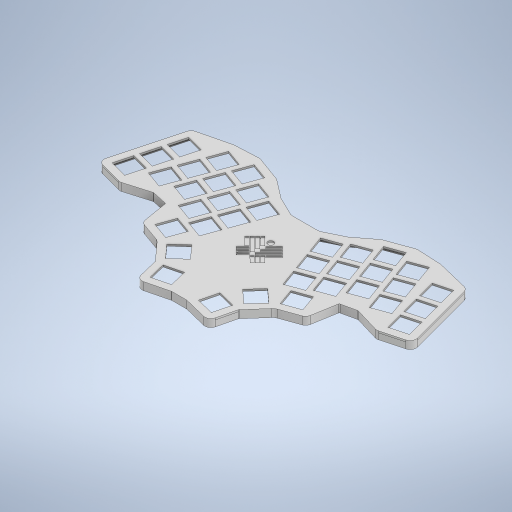
# Autodesk Inventor part: top
Saved by Autodesk Inventor 2024 (Build 280153000, 153)
## iProperties
Created: 2024-10-27
Part Number: top
Material: Generisch
Document SubType Name: Modeling
Designer: nikla
Density: 1 g/cm^3
Appearance: Vorgabe
Author: nikla
Autodesk Inventor part; units mm, degrees
(part 1 of 2)
ref_plane "YZ Plane" through (0, 0, 0) normal (1, 0, 0) x (0, 1, 0)
ref_plane "XZ Plane" through (0, 0, 0) normal (0, 1, 0) x (-1, 0, 0)
ref_plane "XY Plane" through (0, 0, 0) normal (0, 0, 1) x (1, 0, 0)
sketch "Skizze3" plane through (0, 0, 0) normal (0, 0, 1) x (1, 0, 0)
  line L0 (33.2927, 55.6855) -> (15.6286, 55.6855) projected
  line L1 (11.8229, 56.0361) -> (-3.9316, 63.7231) projected
  line L2 (37.0985, 56.0361) -> (52.8529, 63.7231) projected
  arc A0 (69.5641, 76.2372) -> (68.2289, 75.5042) centre (71.2739, 71.5396) ccw projected
  arc A1 (91.9431, 83.9654) -> (89.9858, 83.67) centre (91.6959, 78.9716) ccw projected
  arc A2 (112.5928, 82.8509) -> (111.6421, 82.9904) centre (111.3949, 77.9956) ccw projected
  arc A3 (141.8721, 73.0196) -> (138.2304, 76.582) centre (137.0429, 71.7256) ccw projected
  line L3 (141.8721, 73.0196) -> (156.3724, 18.9046) projected
  arc A4 (152.837, 12.781) -> (156.3724, 18.9046) centre (151.5429, 17.6106) ccw projected
  line L4 (152.837, 12.781) -> (134.5249, 7.8743) projected
  line L5 (131.8222, 7.9065) -> (111.3881, 13.9074) projected
  arc A5 (131.8222, 7.9065) -> (134.5249, 7.8743) centre (133.2309, 12.7036) ccw projected
  line L6 (110.8785, 13.9276) -> (98.6315, 11.2116) projected
  line L7 (97.8626, 10.4048) -> (94.4059, -9.7209) projected
  line L8 (91.1608, -13.5829) -> (75.8602, -19.0515) projected
  line L9 (59.9635, -35.5881) -> (72.8683, -21.2559) projected
  line L10 (55.8813, -51.867) -> (59.7317, -36.0348) projected
  line L11 (30.9758, -50.8402) -> (49.8133, -55.5369) projected
  arc A6 (49.8133, -55.5369) -> (55.8813, -51.867) centre (51.0229, -50.6854) ccw projected
  line L12 (18.202, -50.8106) -> (30.7193, -50.8106) projected
  line L13 (-0.892, -55.5369) -> (17.9455, -50.8402) projected
  arc A7 (-6.96, -51.867) -> (-0.892, -55.5369) centre (-2.1016, -50.6854) ccw projected
  line L14 (-10.8104, -36.0348) -> (-6.96, -51.867) projected
  line L15 (-23.947, -21.2559) -> (-11.0422, -35.5881) projected
  line L16 (-42.2395, -13.5829) -> (-26.9389, -19.0515) projected
  line L17 (-48.9413, 10.4048) -> (-45.4846, -9.7209) projected
  arc A8 (-45.4846, -9.7209) -> (-42.2395, -13.5829) centre (-40.5566, -8.8744) ccw projected
  line L18 (-61.9572, 13.9276) -> (-49.7102, 11.2116) projected
  line L19 (-82.9009, 7.9065) -> (-62.4668, 13.9074) projected
  line L20 (-103.9157, 12.781) -> (-85.6036, 7.8743) projected
  arc A9 (-107.4511, 18.9046) -> (-103.9157, 12.781) centre (-102.6216, 17.6106) ccw projected
  line L21 (-92.9508, 73.0196) -> (-107.4511, 18.9046) projected
  line L22 (-63.6715, 82.8509) -> (-89.3091, 76.582) projected
  arc A10 (-89.3091, 76.582) -> (-92.9508, 73.0196) centre (-88.1216, 71.7256) ccw projected
  line L23 (-4.112, 63.8334) -> (-19.3076, 75.5043) projected
  line L24 (-20.6428, 76.2372) -> (-41.0645, 83.67) projected
  line L25 (-43.0218, 83.9654) -> (-62.7208, 82.9904) projected
  line L26 (53.0333, 63.8334) -> (68.2289, 75.5043) projected
  line L27 (69.5641, 76.2372) -> (89.9858, 83.67) projected
  line L28 (91.9431, 83.9654) -> (111.6421, 82.9904) projected
  line L29 (112.5928, 82.8509) -> (138.2304, 76.582) projected
  line L30 (-82.1125, 32.7172) -> (-96.6013, 36.5996) projected
  line L31 (-96.6013, 36.5996) -> (-92.719, 51.0885) projected
  line L32 (-92.719, 51.0885) -> (-78.2301, 47.2061) projected
  line L33 (-78.2301, 47.2061) -> (-82.1125, 32.7172) projected
  line L34 (-31.0217, 57.7735) -> (-45.117, 62.9038) projected
  line L35 (-45.117, 62.9038) -> (-39.9867, 76.9992) projected
  line L36 (-39.9867, 76.9992) -> (-25.8914, 71.8689) projected
  line L37 (-25.8914, 71.8689) -> (-31.0217, 57.7735) projected
  line L38 (-16.5877, 41.8782) -> (-21.718, 27.7828) projected
  line L39 (-21.718, 27.7828) -> (-35.8134, 32.9131) projected
  line L40 (-35.8134, 32.9131) -> (-30.6831, 47.0085) projected
  line L41 (-30.6831, 47.0085) -> (-16.5877, 41.8782) projected
  line L42 (-20.0113, 20.7765) -> (-5.916, 15.6462) projected
  line L43 (-5.916, 15.6462) -> (-11.0463, 1.5508) projected
  line L44 (-11.0463, 1.5508) -> (-25.1417, 6.6811) projected
  line L45 (-25.1417, 6.6811) -> (-20.0113, 20.7765) projected
  line L46 (-4.5479, 19.405) -> (-18.6433, 24.5353) projected
  line L47 (-18.6433, 24.5353) -> (-13.513, 38.6307) projected
  line L48 (-13.513, 38.6307) -> (0.5824, 33.5004) projected
  line L49 (0.5824, 33.5004) -> (-4.5479, 19.405) projected
  line L50 (-10.0893, 59.7323) -> (-15.2196, 45.6369) projected
  line L51 (-15.2196, 45.6369) -> (-29.315, 50.7672) projected
  line L52 (-29.315, 50.7672) -> (-24.1847, 64.8626) projected
  line L53 (-24.1847, 64.8626) -> (-10.0893, 59.7323) projected
  line L54 (-59.4784, 35.1414) -> (-64.6087, 21.046) projected
  line L55 (-64.6087, 21.046) -> (-78.7041, 26.1763) projected
  line L56 (-78.7041, 26.1763) -> (-73.5738, 40.2717) projected
  line L57 (-73.5738, 40.2717) -> (-59.4784, 35.1414) projected
  line L58 (-77.1948, 51.0698) -> (-91.6837, 54.9522) projected
  line L59 (-91.6837, 54.9522) -> (-87.8013, 69.441) projected
  line L60 (-87.8013, 69.441) -> (-73.3125, 65.5587) projected
  line L61 (-73.3125, 65.5587) -> (-77.1948, 51.0698) projected
  line L62 (-46.4817, 70.8497) -> (-51.612, 56.7543) projected
  line L63 (-51.612, 56.7543) -> (-65.7074, 61.8846) projected
  line L64 (-65.7074, 61.8846) -> (-60.5771, 75.98) projected
  line L65 (-60.5771, 75.98) -> (-46.4817, 70.8497) projected
  line L66 (-37.52, 39.9193) -> (-51.6154, 45.0496) projected
  line L67 (-51.6154, 45.0496) -> (-46.4851, 59.145) projected
  line L68 (-46.4851, 59.145) -> (-32.3897, 54.0147) projected
  line L69 (-32.3897, 54.0147) -> (-37.52, 39.9193) projected
  line L70 (-37.1815, 29.1543) -> (-23.0861, 24.024) projected
  line L71 (-23.0861, 24.024) -> (-28.2164, 9.9286) projected
  line L72 (-28.2164, 9.9286) -> (-42.3118, 15.0589) projected
  line L73 (-42.3118, 15.0589) -> (-37.1815, 29.1543) projected
  line L74 (-33.1433, 5.2903) -> (-19.0184, 0.2419) projected
  line L75 (-19.0184, 0.2419) -> (-24.0668, -13.883) projected
  line L76 (-24.0668, -13.883) -> (-38.1917, -8.8346) projected
  line L77 (-38.1917, -8.8346) -> (-33.1433, 5.2903) projected
  line L78 (1.9505, 37.2592) -> (-12.1449, 42.3895) projected
  line L79 (-12.1449, 42.3895) -> (-7.0146, 56.4848) projected
  line L80 (-7.0146, 56.4848) -> (7.0808, 51.3545) projected
  line L81 (7.0808, 51.3545) -> (1.9505, 37.2592) projected
  line L82 (-52.9835, 41.2908) -> (-38.8881, 36.1605) projected
  line L83 (-38.8881, 36.1605) -> (-44.0184, 22.0651) projected
  line L84 (-44.0184, 22.0651) -> (-58.1138, 27.1954) projected
  line L85 (-58.1138, 27.1954) -> (-52.9835, 41.2908) projected
  line L86 (-52.9801, 52.9955) -> (-58.1104, 38.9001) projected
  line L87 (-58.1104, 38.9001) -> (-72.2057, 44.0304) projected
  line L88 (-72.2057, 44.0304) -> (-67.0754, 58.1258) projected
  line L89 (-67.0754, 58.1258) -> (-52.9801, 52.9955) projected
  line L90 (-97.6366, 32.7359) -> (-83.1478, 28.8535) projected
  line L91 (-83.1478, 28.8535) -> (-87.0301, 14.3647) projected
  line L92 (-87.0301, 14.3647) -> (-101.519, 18.247) projected
  line L93 (-101.519, 18.247) -> (-97.6366, 32.7359) projected
  arc A11 (-85.086, 9.8061) -> (-83.4644, 9.8255) centre (-84.3096, 12.7036) ccw projected
  line L94 (-63.0418, 15.823) -> (-83.4644, 9.8255) projected
  arc A12 (-61.5241, 15.8802) -> (-63.0418, 15.8229) centre (-62.1736, 12.9516) ccw projected
  line L95 (-49.2771, 13.1641) -> (-61.5241, 15.8802) projected
  arc A13 (-46.9702, 10.7433) -> (-49.2771, 13.1641) centre (-49.9266, 10.2356) ccw projected
  line L96 (-43.5135, -9.3823) -> (-46.9702, 10.7433) projected
  arc A14 (-43.5135, -9.3823) -> (-41.5663, -11.6996) centre (-40.5566, -8.8744) ccw projected
  line L97 (-26.2657, -17.1682) -> (-41.5663, -11.6996) projected
  arc A15 (-26.2657, -17.1682) -> (-25.1373, -16.9454) centre (-25.8881, -16.1115) ccw projected
  line L98 (-10.1529, -3.4534) -> (-25.1373, -16.9454) projected
  line L99 (10.8605, 54.2803) -> (-10.1529, -3.4534) projected
  line L100 (-4.7986, 61.9207) -> (10.8605, 54.2803) projected
  arc A16 (-5.3302, 62.2473) -> (-4.7986, 61.9208) centre (-3.5036, 64.6256) ccw projected
  line L101 (-20.5258, 73.9181) -> (-5.3302, 62.2473) projected
  arc A17 (-20.5258, 73.9181) -> (-21.3269, 74.3578) centre (-22.3526, 71.5396) ccw projected
  line L102 (-41.7486, 81.7906) -> (-21.3269, 74.3578) projected
  arc A18 (-41.7486, 81.7906) -> (-42.9229, 81.9679) centre (-42.7746, 78.9716) ccw projected
  line L103 (-62.622, 80.9928) -> (-42.9229, 81.9679) projected
  arc A19 (-62.622, 80.9928) -> (-63.1944, 80.9086) centre (-62.4736, 77.9956) ccw projected
  line L104 (-88.8341, 74.6393) -> (-63.1944, 80.9086) projected
  arc A20 (-88.8341, 74.6393) -> (-91.019, 72.5019) centre (-88.1216, 71.7256) ccw projected
  line L105 (-105.5193, 18.387) -> (-91.019, 72.5019) projected
  arc A21 (-105.5193, 18.387) -> (-103.398, 14.7129) centre (-102.6216, 17.6106) ccw projected
  line L106 (-85.086, 9.8061) -> (-103.398, 14.7129) projected
  line L107 (131.0338, 32.7172) -> (145.5226, 36.5996) projected
  line L108 (127.1514, 47.2061) -> (131.0338, 32.7172) projected
  line L109 (141.6403, 51.0885) -> (127.1514, 47.2061) projected
  line L110 (145.5226, 36.5996) -> (141.6403, 51.0885) projected
  line L111 (79.943, 57.7735) -> (94.0383, 62.9038) projected
  line L112 (74.8127, 71.8689) -> (79.943, 57.7735) projected
  line L113 (88.908, 76.9992) -> (74.8127, 71.8689) projected
  line L114 (94.0383, 62.9038) -> (88.908, 76.9992) projected
  line L115 (65.509, 41.8782) -> (70.6393, 27.7828) projected
  line L116 (79.6044, 47.0085) -> (65.509, 41.8782) projected
  line L117 (84.7347, 32.9131) -> (79.6044, 47.0085) projected
  line L118 (70.6393, 27.7828) -> (84.7347, 32.9131) projected
  line L119 (68.9327, 20.7765) -> (54.8373, 15.6462) projected
  line L120 (74.063, 6.6811) -> (68.9327, 20.7765) projected
  line L121 (59.9676, 1.5508) -> (74.063, 6.6811) projected
  line L122 (54.8373, 15.6462) -> (59.9676, 1.5508) projected
  line L123 (53.4692, 19.405) -> (67.5646, 24.5353) projected
  line L124 (48.3389, 33.5004) -> (53.4692, 19.405) projected
  line L125 (62.4343, 38.6307) -> (48.3389, 33.5004) projected
  line L126 (67.5646, 24.5353) -> (62.4343, 38.6307) projected
  line L127 (59.0106, 59.7323) -> (64.1409, 45.6369) projected
  line L128 (73.106, 64.8626) -> (59.0106, 59.7323) projected
  line L129 (78.2363, 50.7672) -> (73.106, 64.8626) projected
  line L130 (64.1409, 45.6369) -> (78.2363, 50.7672) projected
  line L131 (108.3997, 35.1414) -> (113.53, 21.046) projected
  line L132 (122.4951, 40.2717) -> (108.3997, 35.1414) projected
  line L133 (127.6254, 26.1763) -> (122.4951, 40.2717) projected
  line L134 (113.53, 21.046) -> (127.6254, 26.1763) projected
  line L135 (126.1161, 51.0698) -> (140.605, 54.9522) projected
  line L136 (122.2338, 65.5587) -> (126.1161, 51.0698) projected
  line L137 (136.7226, 69.441) -> (122.2338, 65.5587) projected
  line L138 (140.605, 54.9522) -> (136.7226, 69.441) projected
  line L139 (95.403, 70.8497) -> (100.5333, 56.7543) projected
  line L140 (109.4984, 75.98) -> (95.403, 70.8497) projected
  line L141 (114.6287, 61.8846) -> (109.4984, 75.98) projected
  line L142 (100.5333, 56.7543) -> (114.6287, 61.8846) projected
  line L143 (86.4413, 39.9193) -> (100.5367, 45.0496) projected
  line L144 (81.311, 54.0147) -> (86.4413, 39.9193) projected
  line L145 (95.4064, 59.145) -> (81.311, 54.0147) projected
  line L146 (100.5367, 45.0496) -> (95.4064, 59.145) projected
  line L147 (86.1028, 29.1543) -> (72.0074, 24.024) projected
  line L148 (91.2331, 15.0589) -> (86.1028, 29.1543) projected
  line L149 (77.1377, 9.9286) -> (91.2331, 15.0589) projected
  line L150 (72.0074, 24.024) -> (77.1377, 9.9286) projected
  line L151 (82.0646, 5.2903) -> (67.9397, 0.2419) projected
  line L152 (87.113, -8.8346) -> (82.0646, 5.2903) projected
  line L153 (72.9881, -13.883) -> (87.113, -8.8346) projected
  line L154 (67.9397, 0.2419) -> (72.9881, -13.883) projected
  line L155 (46.9708, 37.2592) -> (61.0662, 42.3895) projected
  line L156 (41.8405, 51.3545) -> (46.9708, 37.2592) projected
  line L157 (55.9359, 56.4848) -> (41.8405, 51.3545) projected
  line L158 (61.0662, 42.3895) -> (55.9359, 56.4848) projected
  line L159 (101.9048, 41.2908) -> (87.8094, 36.1605) projected
  line L160 (107.0351, 27.1954) -> (101.9048, 41.2908) projected
  line L161 (92.9397, 22.0651) -> (107.0351, 27.1954) projected
  line L162 (87.8094, 36.1605) -> (92.9397, 22.0651) projected
  line L163 (101.9014, 52.9955) -> (107.0317, 38.9001) projected
  line L164 (115.9967, 58.1258) -> (101.9014, 52.9955) projected
  line L165 (121.1271, 44.0304) -> (115.9967, 58.1258) projected
  line L166 (107.0317, 38.9001) -> (121.1271, 44.0304) projected
  line L167 (146.5579, 32.7359) -> (132.0691, 28.8535) projected
  line L168 (150.4403, 18.247) -> (146.5579, 32.7359) projected
  line L169 (135.9514, 14.3647) -> (150.4403, 18.247) projected
  line L170 (132.0691, 28.8535) -> (135.9514, 14.3647) projected
  arc A22 (132.3857, 9.8255) -> (134.0073, 9.8061) centre (133.2309, 12.7036) ccw projected
  line L171 (134.0073, 9.8061) -> (152.3194, 14.7129) projected
  arc A23 (152.3194, 14.7129) -> (154.4406, 18.387) centre (151.5429, 17.6106) ccw projected
  line L172 (154.4406, 18.387) -> (139.9403, 72.5019) projected
  arc A24 (139.9403, 72.5019) -> (137.7554, 74.6393) centre (137.0429, 71.7256) ccw projected
  line L173 (137.7554, 74.6393) -> (112.1157, 80.9086) projected
  arc A25 (112.1157, 80.9086) -> (111.5433, 80.9928) centre (111.3949, 77.9956) ccw projected
  line L174 (111.5433, 80.9928) -> (91.8442, 81.9679) projected
  arc A26 (91.8442, 81.9679) -> (90.6699, 81.7906) centre (91.6959, 78.9716) ccw projected
  line L175 (90.6699, 81.7906) -> (70.2482, 74.3578) projected
  arc A27 (70.2482, 74.3578) -> (69.4471, 73.9181) centre (71.2739, 71.5396) ccw projected
  line L176 (69.4471, 73.9181) -> (54.2515, 62.2473) projected
  arc A28 (53.7199, 61.9208) -> (54.2515, 62.2473) centre (52.4249, 64.6256) ccw projected
  line L177 (53.7199, 61.9207) -> (38.0608, 54.2803) projected
  line L178 (38.0608, 54.2803) -> (59.0742, -3.4534) projected
  line L179 (59.0742, -3.4534) -> (74.0586, -16.9454) projected
  arc A29 (74.0586, -16.9454) -> (75.187, -17.1682) centre (74.8094, -16.1115) ccw projected
  line L180 (75.187, -17.1682) -> (90.4877, -11.6996) projected
  arc A30 (90.4877, -11.6996) -> (92.4348, -9.3823) centre (89.4779, -8.8744) ccw projected
  line L181 (92.4348, -9.3823) -> (95.8915, 10.7433) projected
  arc A31 (98.1984, 13.1641) -> (95.8915, 10.7433) centre (98.8479, 10.2356) ccw projected
  line L182 (98.1984, 13.1641) -> (110.4454, 15.8802) projected
  arc A32 (111.9631, 15.8229) -> (110.4454, 15.8802) centre (111.0949, 12.9516) ccw projected
  line L183 (111.9631, 15.823) -> (132.3857, 9.8255) projected
  line L184 (-18.7976, -18.1574) -> (-7.6504, -8.1205) projected
  line L185 (-7.6504, -8.1205) -> (2.3865, -19.2676) projected
  line L186 (2.3865, -19.2676) -> (-8.7607, -29.3046) projected
  line L187 (-8.7607, -29.3046) -> (-18.7976, -18.1574) projected
  line L188 (-5.0923, -35.0444) -> (9.4622, -31.4155) projected
  line L189 (9.4622, -31.4155) -> (13.091, -45.97) projected
  line L190 (13.091, -45.97) -> (-1.4635, -49.5988) projected
  line L191 (-1.4635, -49.5988) -> (-5.0923, -35.0444) projected
  line L192 (56.5717, -8.1205) -> (67.7189, -18.1574) projected
  line L193 (67.7189, -18.1574) -> (57.682, -29.3046) projected
  line L194 (57.682, -29.3046) -> (46.5348, -19.2676) projected
  line L195 (46.5348, -19.2676) -> (56.5717, -8.1205) projected
  line L196 (39.4592, -31.4155) -> (54.0136, -35.0444) projected
  line L197 (54.0136, -35.0444) -> (50.3848, -49.5988) projected
  line L198 (50.3848, -49.5988) -> (35.8303, -45.97) projected
  line L199 (35.8303, -45.97) -> (39.4592, -31.4155) projected
  line L200 (40.3585, 20.6367) -> (33.3036, 13.605) projected
  line L201 (33.3036, 13.605) -> (31.4884, 15.4262) projected
  line L202 (31.4884, 15.4262) -> (38.5432, 22.458) projected
  line L203 (38.5432, 22.458) -> (40.3585, 20.6367) projected
  line L204 (32.0676, 5.1044) -> (30.2744, 3.2872) projected
  line L205 (30.2744, 3.2872) -> (24.8042, 8.6849) projected
  line L206 (24.8042, 8.6849) -> (26.5973, 10.5022) projected
  line L207 (26.5973, 10.5022) -> (32.0676, 5.1044) projected
  line L208 (38.1322, 22.8703) -> (26.5571, 11.3331) projected
  line L209 (26.5571, 11.3331) -> (24.7508, 13.1453) projected
  line L210 (24.7508, 13.1453) -> (36.3259, 24.6825) projected
  line L211 (36.3259, 24.6825) -> (38.1322, 22.8703) projected
  line L212 (33.696, 27.342) -> (26.6365, 20.2085) projected
  line L213 (26.6365, 20.2085) -> (24.8042, 22.0219) projected
  line L214 (24.8042, 22.0219) -> (31.8637, 29.1553) projected
  line L215 (31.8637, 29.1553) -> (33.696, 27.342) projected
  line L216 (36.5038, 9.5173) -> (34.662, 7.6816) projected
  line L217 (34.662, 7.6816) -> (29.2081, 13.1534) projected
  line L218 (29.2081, 13.1534) -> (31.0499, 14.9892) projected
  line L219 (31.0499, 14.9892) -> (36.5038, 9.5173) projected
  line L220 (34.2705, 7.2913) -> (32.422, 5.4489) projected
  line L221 (32.422, 5.4489) -> (26.9681, 10.9208) projected
  line L222 (26.9681, 10.9208) -> (28.8165, 12.7631) projected
  line L223 (28.8165, 12.7631) -> (34.2705, 7.2913) projected
  line L224 (35.9113, 25.0985) -> (26.5762, 15.7939) projected
  line L225 (26.5762, 15.7939) -> (24.7642, 17.6119) projected
  line L226 (24.7642, 17.6119) -> (34.0993, 26.9165) projected
  line L227 (34.0993, 26.9165) -> (35.9113, 25.0985) projected
  line L228 (15.6177, 13.605) -> (8.5628, 20.6367) projected
  line L229 (8.5628, 20.6367) -> (10.3781, 22.458) projected
  line L230 (10.3781, 22.458) -> (17.4329, 15.4262) projected
  line L231 (17.4329, 15.4262) -> (15.6177, 13.605) projected
  line L232 (18.6469, 3.2872) -> (16.8537, 5.1044) projected
  line L233 (16.8537, 5.1044) -> (22.324, 10.5022) projected
  line L234 (22.324, 10.5022) -> (24.1171, 8.6849) projected
  line L235 (24.1171, 8.6849) -> (18.6469, 3.2872) projected
  line L236 (22.3642, 11.3331) -> (10.7891, 22.8703) projected
  line L237 (10.7891, 22.8703) -> (12.5954, 24.6825) projected
  line L238 (12.5954, 24.6825) -> (24.1705, 13.1453) projected
  line L239 (24.1705, 13.1453) -> (22.3642, 11.3331) projected
  line L240 (22.2848, 20.2085) -> (15.2253, 27.342) projected
  line L241 (15.2253, 27.342) -> (17.0576, 29.1553) projected
  line L242 (17.0576, 29.1553) -> (24.1171, 22.0219) projected
  line L243 (24.1171, 22.0219) -> (22.2848, 20.2085) projected
  line L244 (14.2593, 7.6816) -> (12.4175, 9.5173) projected
  line L245 (12.4175, 9.5173) -> (17.8714, 14.9892) projected
  line L246 (17.8714, 14.9892) -> (19.7132, 13.1534) projected
  line L247 (19.7132, 13.1534) -> (14.2593, 7.6816) projected
  line L248 (16.4993, 5.4489) -> (14.6508, 7.2913) projected
  line L249 (14.6508, 7.2913) -> (20.1048, 12.7631) projected
  line L250 (20.1048, 12.7631) -> (21.9532, 10.9208) projected
  line L251 (21.9532, 10.9208) -> (16.4993, 5.4489) projected
  line L252 (22.3451, 15.7939) -> (13.01, 25.0985) projected
  line L253 (13.01, 25.0985) -> (14.822, 26.9165) projected
  line L254 (14.822, 26.9165) -> (24.1571, 17.6119) projected
  line L255 (24.1571, 17.6119) -> (22.3451, 15.7939) projected
  circle A33 centre (24.4607, 26.6625) radius 2.4143 projected
  line L256 (-22.4605, -19.9178) -> (-6.7352, -5.7586) projected
  line L257 (-9.5559, -34.2498) -> (-22.4605, -19.9178) projected
  arc A34 (-8.8645, -35.5723) -> (-9.5559, -34.2498) centre (-11.7856, -36.2574) ccw projected
  line L258 (-5.0167, -51.3944) -> (-8.8645, -35.5723) projected
  arc A35 (-5.0167, -51.3944) -> (-1.3758, -53.5964) centre (-2.1016, -50.6854) ccw projected
  line L259 (17.4616, -48.8996) -> (-1.3758, -53.5964) projected
  arc A36 (18.2126, -48.8106) -> (17.4616, -48.8996) centre (18.1874, -51.8104) ccw projected
  line L260 (30.7087, -48.8106) -> (18.2126, -48.8106) projected
  arc A37 (31.4597, -48.8996) -> (30.7087, -48.8106) centre (30.7339, -51.8104) ccw projected
  line L261 (50.2971, -53.5964) -> (31.4597, -48.8996) projected
  arc A38 (50.2971, -53.5964) -> (53.938, -51.3944) centre (51.0229, -50.6854) ccw projected
  line L262 (57.7859, -35.5723) -> (53.938, -51.3944) projected
  arc A39 (58.4772, -34.2498) -> (57.7859, -35.5723) centre (60.7069, -36.2574) ccw projected
  line L263 (71.3818, -19.9178) -> (58.4772, -34.2498) projected
  line L264 (55.6565, -5.7586) -> (71.3818, -19.9178) projected
  line L265 (34.2696, 53.0014) -> (55.6565, -5.7586) projected
  arc A40 (34.2696, 53.0014) -> (33.2927, 53.6855) centre (33.2927, 52.6459) ccw projected
  line L266 (15.6286, 53.6855) -> (33.2927, 53.6855) projected
  arc A41 (15.6286, 53.6855) -> (14.6517, 53.0014) centre (15.6286, 52.6459) ccw projected
  line L267 (-6.7352, -5.7586) -> (14.6517, 53.0014) projected
  line L268 (15.6286, 55.6855) -> (33.2927, 55.6855)
  arc A42 (33.2927, 55.6855) -> (37.0985, 56.0361) centre (33.2927, 76.5174) ccw
  line L269 (37.0985, 56.0361) -> (52.8529, 63.7231)
  line L270 (52.8529, 63.7231) -> (68.2289, 75.5043)
  arc A43 (69.5641, 76.2372) -> (68.2289, 75.5043) centre (71.2739, 71.5395) ccw
  line L271 (69.5641, 76.2372) -> (89.9858, 83.67)
  arc A44 (91.9431, 83.9654) -> (89.9858, 83.67) centre (91.6959, 78.9715) ccw
  line L272 (91.9431, 83.9654) -> (111.5433, 82.9953)
  arc A45 (112.5928, 82.8509) -> (111.5433, 82.9953) centre (111.2427, 76.9229) ccw
  line L273 (112.5928, 82.8509) -> (138.2304, 76.582)
  arc A46 (141.8721, 73.0196) -> (138.2304, 76.582) centre (137.0429, 71.7256) ccw
  line L274 (141.8721, 73.0196) -> (156.3724, 18.9046)
  arc A47 (152.837, 12.781) -> (156.3724, 18.9046) centre (151.5429, 17.6106) ccw
  line L275 (152.837, 12.781) -> (134.5249, 7.8743)
  arc A48 (131.9369, 7.8743) -> (134.5249, 7.8743) centre (133.2309, 12.7036) ccw
  line L276 (131.9369, 7.8743) -> (111.3881, 13.9074)
  arc A49 (111.3881, 13.9074) -> (110.8785, 13.9276) centre (111.093, 12.9022) ccw
  line L277 (110.8785, 13.9276) -> (98.6315, 11.2116)
  arc A50 (98.6315, 11.2116) -> (97.8626, 10.4048) centre (98.8479, 10.2356) ccw
  line L278 (97.8626, 10.4048) -> (94.4059, -9.7209)
  arc A51 (91.1608, -13.5829) -> (94.4059, -9.7209) centre (89.4779, -8.8744) ccw
  line L279 (91.1608, -13.5829) -> (75.8602, -19.0515)
  arc A52 (75.8602, -19.0515) -> (72.8683, -21.2559) centre (78.0345, -25.135) ccw
  line L280 (72.8683, -21.2559) -> (59.9635, -35.5881)
  arc A53 (59.9635, -35.5881) -> (59.7317, -36.0348) centre (60.7069, -36.2574) ccw
  line L281 (59.7317, -36.0348) -> (55.8813, -51.867)
  arc A54 (49.8133, -55.5369) -> (55.8813, -51.867) centre (51.0229, -50.6854) ccw
  line L282 (49.8133, -55.5369) -> (30.9758, -50.8402)
  arc A55 (30.9758, -50.8402) -> (30.7193, -50.8106) centre (30.7339, -51.8104) ccw
  line L283 (30.7193, -50.8106) -> (18.202, -50.8106)
  arc A56 (18.202, -50.8106) -> (17.9455, -50.8402) centre (18.202, -51.9367) ccw
  line L284 (17.9455, -50.8402) -> (-0.892, -55.5369)
  arc A57 (-6.96, -51.867) -> (-0.92, -55.5439) centre (-2.1015, -50.6854) ccw
  line L285 (-6.96, -51.867) -> (-10.8104, -36.0348)
  arc A58 (-10.8104, -36.0348) -> (-11.0422, -35.5881) centre (-11.8384, -36.2849) ccw
  line L286 (-11.0422, -35.5881) -> (-23.919, -21.287)
  arc A59 (-23.919, -21.287) -> (-26.9389, -19.0515) centre (-30.9283, -27.5982) ccw
  line L287 (-26.9389, -19.0515) -> (-42.2395, -13.5829)
  arc A60 (-45.4846, -9.7209) -> (-42.2395, -13.5829) centre (-40.5566, -8.8744) ccw
  line L288 (-45.4846, -9.7209) -> (-48.9413, 10.4048)
  arc A61 (-48.9413, 10.4048) -> (-49.7102, 11.2116) centre (-49.9266, 10.2356) ccw
  line L289 (-49.7102, 11.2116) -> (-61.9572, 13.9276)
  arc A62 (-61.9572, 13.9276) -> (-62.4668, 13.9074) centre (-62.1736, 12.9516) ccw
  line L290 (-62.4668, 13.9074) -> (-82.9009, 7.9065)
  arc A63 (-85.6036, 7.8743) -> (-82.9009, 7.9065) centre (-84.3096, 12.7035) ccw
  line L291 (-85.6036, 7.8743) -> (-103.9157, 12.781)
  arc A64 (-107.4511, 18.9046) -> (-103.9157, 12.781) centre (-102.6216, 17.6106) ccw
  line L292 (-107.4511, 18.9046) -> (-92.9511, 73.0185)
  arc A65 (-89.3091, 76.582) -> (-92.9511, 73.0185) centre (-88.1201, 71.724) ccw
  line L293 (-89.3091, 76.582) -> (-63.6715, 82.8509)
  arc A66 (-62.7208, 82.9904) -> (-63.6715, 82.8509) centre (-62.4577, 77.8869) ccw
  line L294 (-62.7208, 82.9904) -> (-43.0218, 83.9654)
  arc A67 (-41.0645, 83.67) -> (-43.0218, 83.9654) centre (-42.7746, 78.9715) ccw
  line L295 (-41.0645, 83.67) -> (-20.6437, 76.2377)
  arc A68 (-19.3076, 75.5043) -> (-20.6437, 76.2377) centre (-22.3546, 71.5369) ccw
  line L296 (-19.3076, 75.5043) -> (-4.112, 63.8334)
  line L297 (-4.112, 63.8334) -> (-3.7919, 63.6549)
  line L298 (-3.7919, 63.6549) -> (11.8229, 56.0361)
  arc A69 (11.8229, 56.0361) -> (15.6286, 55.6855) centre (15.6286, 76.5174) ccw
  point P0 (0, 0)
  constraints: 62 end point, 57 point on circle, 47 tangent, 28 centre point, 13 collinear, 8 point on line, 1 concentric, 1 horizontal, 1 other
extrude "Extrusion2" add sketch "Skizze3" against normal blind 1.5 contours A42 L2 L270 A0 L27 A1 L28 A2 L29 A3 L3 A4 L4 A5 L5 A49 L6 A50 L7 A51 L8 A52 L9 A53 L10 A6 L11 A55 L12 A56 L13 A7 L14 A58 L15 A59 L16 A8 L17 A61 L18 A62 L19 A63 L20 A9 L21 A10 L22 A66 L25 A67 L24 A68 L23 L297 L1 A69 L0 | L106 A21 L105 A20 L104 A19 L103 A18 L102 A17 L101 A16 L100 L99 L98 A15 L97 A14 L96 A13 L95 A12 L94 A11 | L183 A32 L182 A31 L181 A30 L180 A29 L179 L178 L177 A28 L176 A27 L175 A26 L174 A25 L173 A24 L172 A23 L171 A22 | L256 L267 A41 L266 A40 L265 L264 L263 A39 L262 A38 L261 A37 L260 A36 L259 A35 L258 A34 L257
sketch "Skizze5" plane through (0, 0, -1.5) normal (0, 0, -1) x (-1, 0, 0)
  line L0 (-131.9369, 7.8743) -> (-111.3881, 13.9074) projected
  arc A0 (-110.8785, 13.9276) -> (-111.3881, 13.9074) centre (-111.093, 12.9022) ccw projected
  line L1 (-110.8785, 13.9276) -> (-98.6315, 11.2116) projected
  arc A1 (-97.8626, 10.4048) -> (-98.6315, 11.2116) centre (-98.8479, 10.2356) ccw projected
  line L2 (-97.8626, 10.4048) -> (-94.4059, -9.7209) projected
  arc A2 (-94.4059, -9.7209) -> (-91.1608, -13.5829) centre (-89.4779, -8.8744) ccw projected
  line L3 (-91.1608, -13.5829) -> (-75.8602, -19.0515) projected
  arc A3 (-72.8683, -21.2559) -> (-75.8602, -19.0515) centre (-78.0345, -25.135) ccw projected
  line L4 (-72.8683, -21.2559) -> (-59.9635, -35.5881) projected
  arc A4 (-59.7317, -36.0348) -> (-59.9635, -35.5881) centre (-60.7069, -36.2574) ccw projected
  line L5 (-59.7317, -36.0348) -> (-55.8813, -51.867) projected
  arc A5 (-55.8813, -51.867) -> (-49.8133, -55.5369) centre (-51.0229, -50.6854) ccw projected
  line L6 (-49.8133, -55.5369) -> (-30.9758, -50.8402) projected
  arc A6 (-30.7193, -50.8106) -> (-30.9758, -50.8402) centre (-30.7339, -51.8104) ccw projected
  line L7 (-30.7193, -50.8106) -> (-18.202, -50.8106) projected
  arc A7 (-17.9455, -50.8402) -> (-18.202, -50.8106) centre (-18.202, -51.9367) ccw projected
  line L8 (-17.9455, -50.8402) -> (0.892, -55.5369) projected
  arc A8 (0.892, -55.5369) -> (6.96, -51.867) centre (2.1016, -50.6854) ccw projected
  line L9 (6.96, -51.867) -> (10.8104, -36.0348) projected
  arc A9 (11.0422, -35.5881) -> (10.8104, -36.0348) centre (11.8384, -36.2849) ccw projected
  line L10 (11.0422, -35.5881) -> (23.919, -21.287) projected
  arc A10 (26.9389, -19.0515) -> (23.919, -21.287) centre (30.9283, -27.5982) ccw projected
  line L11 (26.9389, -19.0515) -> (42.2395, -13.5829) projected
  arc A11 (42.2395, -13.5829) -> (45.4846, -9.7209) centre (40.5566, -8.8744) ccw projected
  line L12 (45.4846, -9.7209) -> (48.9413, 10.4048) projected
  arc A12 (49.7102, 11.2116) -> (48.9413, 10.4048) centre (49.9266, 10.2356) ccw projected
  line L13 (49.7102, 11.2116) -> (61.9572, 13.9276) projected
  arc A13 (62.4668, 13.9074) -> (61.9572, 13.9276) centre (62.1736, 12.9516) ccw projected
  line L14 (62.4668, 13.9074) -> (82.9009, 7.9065) projected
  arc A14 (82.9009, 7.9065) -> (85.6036, 7.8743) centre (84.3096, 12.7035) ccw projected
  line L15 (85.6036, 7.8743) -> (103.9157, 12.781) projected
  arc A15 (103.9157, 12.781) -> (107.4511, 18.9046) centre (102.6216, 17.6106) ccw projected
  line L16 (107.4511, 18.9046) -> (92.9508, 73.0196) projected
  arc A16 (92.9508, 73.0196) -> (89.3091, 76.582) centre (88.1201, 71.724) ccw projected
  line L17 (89.3091, 76.582) -> (63.6715, 82.8509) projected
  arc A17 (63.6715, 82.8509) -> (62.7208, 82.9904) centre (62.4577, 77.8869) ccw projected
  line L18 (62.7208, 82.9904) -> (43.0218, 83.9654) projected
  arc A18 (43.0218, 83.9654) -> (41.0645, 83.67) centre (42.7746, 78.9715) ccw projected
  line L19 (41.0645, 83.67) -> (20.6437, 76.2377) projected
  arc A19 (20.6437, 76.2377) -> (19.3076, 75.5043) centre (22.3546, 71.5369) ccw projected
  line L20 (19.3076, 75.5043) -> (4.112, 63.8334) projected
  line L21 (4.112, 63.8334) -> (3.7919, 63.6549) projected
  line L22 (3.7919, 63.6549) -> (-11.8229, 56.0361) projected
  arc A20 (-15.6286, 55.6855) -> (-11.8229, 56.0361) centre (-15.6286, 76.5174) ccw projected
  line L23 (-15.6286, 55.6855) -> (-33.2927, 55.6855) projected
  arc A21 (-37.0985, 56.0361) -> (-33.2927, 55.6855) centre (-33.2927, 76.5174) ccw projected
  line L24 (-37.0985, 56.0361) -> (-52.8529, 63.7231) projected
  line L25 (-52.8529, 63.7231) -> (-68.2289, 75.5043) projected
  arc A22 (-68.2289, 75.5043) -> (-69.5641, 76.2372) centre (-71.2739, 71.5396) ccw projected
  line L26 (-69.5641, 76.2372) -> (-89.9858, 83.67) projected
  arc A23 (-89.9858, 83.67) -> (-91.9431, 83.9654) centre (-91.6959, 78.9716) ccw projected
  line L27 (-91.9431, 83.9654) -> (-111.5433, 82.9953) projected
  arc A24 (-111.5433, 82.9953) -> (-112.5928, 82.8509) centre (-111.2427, 76.9229) ccw projected
  line L28 (-112.5928, 82.8509) -> (-138.2304, 76.582) projected
  arc A25 (-138.2304, 76.582) -> (-141.8721, 73.0196) centre (-137.0429, 71.7256) ccw projected
  line L29 (-141.8721, 73.0196) -> (-156.3724, 18.9046) projected
  arc A26 (-156.3724, 18.9046) -> (-152.837, 12.781) centre (-151.5429, 17.6106) ccw projected
  line L30 (-152.837, 12.781) -> (-134.5249, 7.8743) projected
  arc A27 (-134.5249, 7.8743) -> (-131.9369, 7.8743) centre (-133.2309, 12.7036) ccw projected
  line L31 (96.6013, 36.5996) -> (82.1125, 32.7172) projected
  line L32 (82.1125, 32.7172) -> (78.2301, 47.2061) projected
  line L33 (78.2301, 47.2061) -> (92.719, 51.0885) projected
  line L34 (92.719, 51.0885) -> (96.6013, 36.5996) projected
  line L35 (45.117, 62.9038) -> (31.0217, 57.7735) projected
  line L36 (31.0217, 57.7735) -> (25.8914, 71.8689) projected
  line L37 (25.8914, 71.8689) -> (39.9867, 76.9992) projected
  line L38 (39.9867, 76.9992) -> (45.117, 62.9038) projected
  line L39 (21.718, 27.7828) -> (16.5877, 41.8782) projected
  line L40 (16.5877, 41.8782) -> (30.6831, 47.0085) projected
  line L41 (30.6831, 47.0085) -> (35.8134, 32.9131) projected
  line L42 (35.8134, 32.9131) -> (21.718, 27.7828) projected
  line L43 (5.916, 15.6462) -> (20.0113, 20.7765) projected
  line L44 (20.0113, 20.7765) -> (25.1417, 6.6811) projected
  line L45 (25.1417, 6.6811) -> (11.0463, 1.5508) projected
  line L46 (11.0463, 1.5508) -> (5.916, 15.6462) projected
  line L47 (18.6433, 24.5353) -> (4.5479, 19.405) projected
  line L48 (4.5479, 19.405) -> (-0.5824, 33.5004) projected
  line L49 (-0.5824, 33.5004) -> (13.513, 38.6307) projected
  line L50 (13.513, 38.6307) -> (18.6433, 24.5353) projected
  line L51 (15.2196, 45.6369) -> (10.0893, 59.7323) projected
  line L52 (10.0893, 59.7323) -> (24.1847, 64.8626) projected
  line L53 (24.1847, 64.8626) -> (29.315, 50.7672) projected
  line L54 (29.315, 50.7672) -> (15.2196, 45.6369) projected
  line L55 (64.6087, 21.046) -> (59.4784, 35.1414) projected
  line L56 (59.4784, 35.1414) -> (73.5738, 40.2717) projected
  line L57 (73.5738, 40.2717) -> (78.7041, 26.1763) projected
  line L58 (78.7041, 26.1763) -> (64.6087, 21.046) projected
  line L59 (91.6837, 54.9522) -> (77.1948, 51.0698) projected
  line L60 (77.1948, 51.0698) -> (73.3125, 65.5587) projected
  line L61 (73.3125, 65.5587) -> (87.8013, 69.441) projected
  line L62 (87.8013, 69.441) -> (91.6837, 54.9522) projected
  line L63 (51.612, 56.7543) -> (46.4817, 70.8497) projected
  line L64 (46.4817, 70.8497) -> (60.5771, 75.98) projected
  line L65 (60.5771, 75.98) -> (65.7074, 61.8846) projected
  line L66 (65.7074, 61.8846) -> (51.612, 56.7543) projected
  line L67 (51.6154, 45.0496) -> (37.52, 39.9193) projected
  line L68 (37.52, 39.9193) -> (32.3897, 54.0147) projected
  line L69 (32.3897, 54.0147) -> (46.4851, 59.145) projected
  line L70 (46.4851, 59.145) -> (51.6154, 45.0496) projected
  line L71 (23.0861, 24.024) -> (37.1815, 29.1543) projected
  line L72 (37.1815, 29.1543) -> (42.3118, 15.0589) projected
  line L73 (42.3118, 15.0589) -> (28.2164, 9.9286) projected
  line L74 (28.2164, 9.9286) -> (23.0861, 24.024) projected
  line L75 (19.0184, 0.2419) -> (33.1433, 5.2903) projected
  line L76 (33.1433, 5.2903) -> (38.1917, -8.8346) projected
  line L77 (38.1917, -8.8346) -> (24.0668, -13.883) projected
  line L78 (24.0668, -13.883) -> (19.0184, 0.2419) projected
  line L79 (12.1449, 42.3895) -> (-1.9505, 37.2592) projected
  line L80 (-1.9505, 37.2592) -> (-7.0808, 51.3545) projected
  line L81 (-7.0808, 51.3545) -> (7.0146, 56.4848) projected
  line L82 (7.0146, 56.4848) -> (12.1449, 42.3895) projected
  line L83 (38.8881, 36.1605) -> (52.9835, 41.2908) projected
  line L84 (52.9835, 41.2908) -> (58.1138, 27.1954) projected
  line L85 (58.1138, 27.1954) -> (44.0184, 22.0651) projected
  line L86 (44.0184, 22.0651) -> (38.8881, 36.1605) projected
  line L87 (58.1104, 38.9001) -> (52.9801, 52.9955) projected
  line L88 (52.9801, 52.9955) -> (67.0754, 58.1258) projected
  line L89 (67.0754, 58.1258) -> (72.2057, 44.0304) projected
  line L90 (72.2057, 44.0304) -> (58.1104, 38.9001) projected
  line L91 (83.1478, 28.8535) -> (97.6366, 32.7359) projected
  line L92 (97.6366, 32.7359) -> (101.519, 18.247) projected
  line L93 (101.519, 18.247) -> (87.0301, 14.3647) projected
  line L94 (87.0301, 14.3647) -> (83.1478, 28.8535) projected
  line L95 (-127.1514, 47.2061) -> (-131.0338, 32.7172) projected
  line L96 (-131.0338, 32.7172) -> (-145.5226, 36.5996) projected
  line L97 (-145.5226, 36.5996) -> (-141.6403, 51.0885) projected
  line L98 (-141.6403, 51.0885) -> (-127.1514, 47.2061) projected
  line L99 (-74.8127, 71.8689) -> (-79.943, 57.7735) projected
  line L100 (-79.943, 57.7735) -> (-94.0383, 62.9038) projected
  line L101 (-94.0383, 62.9038) -> (-88.908, 76.9992) projected
  line L102 (-88.908, 76.9992) -> (-74.8127, 71.8689) projected
  line L103 (-79.6044, 47.0085) -> (-65.509, 41.8782) projected
  line L104 (-65.509, 41.8782) -> (-70.6393, 27.7828) projected
  line L105 (-70.6393, 27.7828) -> (-84.7347, 32.9131) projected
  line L106 (-84.7347, 32.9131) -> (-79.6044, 47.0085) projected
  line L107 (-74.063, 6.6811) -> (-68.9327, 20.7765) projected
  line L108 (-68.9327, 20.7765) -> (-54.8373, 15.6462) projected
  line L109 (-54.8373, 15.6462) -> (-59.9676, 1.5508) projected
  line L110 (-59.9676, 1.5508) -> (-74.063, 6.6811) projected
  line L111 (-48.3389, 33.5004) -> (-53.4692, 19.405) projected
  line L112 (-53.4692, 19.405) -> (-67.5646, 24.5353) projected
  line L113 (-67.5646, 24.5353) -> (-62.4343, 38.6307) projected
  line L114 (-62.4343, 38.6307) -> (-48.3389, 33.5004) projected
  line L115 (-73.106, 64.8626) -> (-59.0106, 59.7323) projected
  line L116 (-59.0106, 59.7323) -> (-64.1409, 45.6369) projected
  line L117 (-64.1409, 45.6369) -> (-78.2363, 50.7672) projected
  line L118 (-78.2363, 50.7672) -> (-73.106, 64.8626) projected
  line L119 (-122.4951, 40.2717) -> (-108.3997, 35.1414) projected
  line L120 (-108.3997, 35.1414) -> (-113.53, 21.046) projected
  line L121 (-113.53, 21.046) -> (-127.6254, 26.1763) projected
  line L122 (-127.6254, 26.1763) -> (-122.4951, 40.2717) projected
  line L123 (-122.2338, 65.5587) -> (-126.1161, 51.0698) projected
  line L124 (-126.1161, 51.0698) -> (-140.605, 54.9522) projected
  line L125 (-140.605, 54.9522) -> (-136.7226, 69.441) projected
  line L126 (-136.7226, 69.441) -> (-122.2338, 65.5587) projected
  line L127 (-109.4984, 75.98) -> (-95.403, 70.8497) projected
  line L128 (-95.403, 70.8497) -> (-100.5333, 56.7543) projected
  line L129 (-100.5333, 56.7543) -> (-114.6287, 61.8846) projected
  line L130 (-114.6287, 61.8846) -> (-109.4984, 75.98) projected
  line L131 (-81.311, 54.0147) -> (-86.4413, 39.9193) projected
  line L132 (-86.4413, 39.9193) -> (-100.5367, 45.0496) projected
  line L133 (-100.5367, 45.0496) -> (-95.4064, 59.145) projected
  line L134 (-95.4064, 59.145) -> (-81.311, 54.0147) projected
  line L135 (-91.2331, 15.0589) -> (-86.1028, 29.1543) projected
  line L136 (-86.1028, 29.1543) -> (-72.0074, 24.024) projected
  line L137 (-72.0074, 24.024) -> (-77.1377, 9.9286) projected
  line L138 (-77.1377, 9.9286) -> (-91.2331, 15.0589) projected
  line L139 (-87.113, -8.8346) -> (-82.0646, 5.2903) projected
  line L140 (-82.0646, 5.2903) -> (-67.9397, 0.2419) projected
  line L141 (-67.9397, 0.2419) -> (-72.9881, -13.883) projected
  line L142 (-72.9881, -13.883) -> (-87.113, -8.8346) projected
  line L143 (-41.8405, 51.3545) -> (-46.9708, 37.2592) projected
  line L144 (-46.9708, 37.2592) -> (-61.0662, 42.3895) projected
  line L145 (-61.0662, 42.3895) -> (-55.9359, 56.4848) projected
  line L146 (-55.9359, 56.4848) -> (-41.8405, 51.3545) projected
  line L147 (-107.0351, 27.1954) -> (-101.9048, 41.2908) projected
  line L148 (-101.9048, 41.2908) -> (-87.8094, 36.1605) projected
  line L149 (-87.8094, 36.1605) -> (-92.9397, 22.0651) projected
  line L150 (-92.9397, 22.0651) -> (-107.0351, 27.1954) projected
  line L151 (-115.9967, 58.1258) -> (-101.9014, 52.9955) projected
  line L152 (-101.9014, 52.9955) -> (-107.0317, 38.9001) projected
  line L153 (-107.0317, 38.9001) -> (-121.1271, 44.0304) projected
  line L154 (-121.1271, 44.0304) -> (-115.9967, 58.1258) projected
  line L155 (-150.4403, 18.247) -> (-146.5579, 32.7359) projected
  line L156 (-146.5579, 32.7359) -> (-132.0691, 28.8535) projected
  line L157 (-132.0691, 28.8535) -> (-135.9514, 14.3647) projected
  line L158 (-135.9514, 14.3647) -> (-150.4403, 18.247) projected
  circle A28 centre (-24.4607, 26.6625) radius 2.4143 projected
  line L159 (-13.01, 25.0985) -> (-22.3451, 15.7939) projected
  line L160 (-22.3451, 15.7939) -> (-24.1571, 17.6119) projected
  line L161 (-24.1571, 17.6119) -> (-14.822, 26.9165) projected
  line L162 (-14.822, 26.9165) -> (-13.01, 25.0985) projected
  line L163 (-14.6508, 7.2913) -> (-16.4993, 5.4489) projected
  line L164 (-16.4993, 5.4489) -> (-21.9532, 10.9208) projected
  line L165 (-21.9532, 10.9208) -> (-20.1048, 12.7631) projected
  line L166 (-20.1048, 12.7631) -> (-14.6508, 7.2913) projected
  line L167 (-12.4175, 9.5173) -> (-14.2593, 7.6816) projected
  line L168 (-14.2593, 7.6816) -> (-19.7132, 13.1534) projected
  line L169 (-19.7132, 13.1534) -> (-17.8714, 14.9892) projected
  line L170 (-17.8714, 14.9892) -> (-12.4175, 9.5173) projected
  line L171 (-15.2253, 27.342) -> (-22.2848, 20.2085) projected
  line L172 (-22.2848, 20.2085) -> (-24.1171, 22.0219) projected
  line L173 (-24.1171, 22.0219) -> (-17.0576, 29.1553) projected
  line L174 (-17.0576, 29.1553) -> (-15.2253, 27.342) projected
  line L175 (-10.7891, 22.8703) -> (-22.3642, 11.3331) projected
  line L176 (-22.3642, 11.3331) -> (-24.1705, 13.1453) projected
  line L177 (-24.1705, 13.1453) -> (-12.5954, 24.6825) projected
  line L178 (-12.5954, 24.6825) -> (-10.7891, 22.8703) projected
  line L179 (-16.8537, 5.1044) -> (-18.6469, 3.2872) projected
  line L180 (-18.6469, 3.2872) -> (-24.1171, 8.6849) projected
  line L181 (-24.1171, 8.6849) -> (-22.324, 10.5022) projected
  line L182 (-22.324, 10.5022) -> (-16.8537, 5.1044) projected
  line L183 (-8.5628, 20.6367) -> (-15.6177, 13.605) projected
  line L184 (-15.6177, 13.605) -> (-17.4329, 15.4262) projected
  line L185 (-17.4329, 15.4262) -> (-10.3781, 22.458) projected
  line L186 (-10.3781, 22.458) -> (-8.5628, 20.6367) projected
  line L187 (-26.5762, 15.7939) -> (-35.9113, 25.0985) projected
  line L188 (-35.9113, 25.0985) -> (-34.0993, 26.9165) projected
  line L189 (-34.0993, 26.9165) -> (-24.7642, 17.6119) projected
  line L190 (-24.7642, 17.6119) -> (-26.5762, 15.7939) projected
  line L191 (-32.422, 5.4489) -> (-34.2705, 7.2913) projected
  line L192 (-34.2705, 7.2913) -> (-28.8165, 12.7631) projected
  line L193 (-28.8165, 12.7631) -> (-26.9681, 10.9208) projected
  line L194 (-26.9681, 10.9208) -> (-32.422, 5.4489) projected
  line L195 (-34.662, 7.6816) -> (-36.5038, 9.5173) projected
  line L196 (-36.5038, 9.5173) -> (-31.0499, 14.9892) projected
  line L197 (-31.0499, 14.9892) -> (-29.2081, 13.1534) projected
  line L198 (-29.2081, 13.1534) -> (-34.662, 7.6816) projected
  line L199 (-26.6365, 20.2085) -> (-33.696, 27.342) projected
  line L200 (-33.696, 27.342) -> (-31.8637, 29.1553) projected
  line L201 (-31.8637, 29.1553) -> (-24.8042, 22.0219) projected
  line L202 (-24.8042, 22.0219) -> (-26.6365, 20.2085) projected
  line L203 (-26.5571, 11.3331) -> (-38.1322, 22.8703) projected
  line L204 (-38.1322, 22.8703) -> (-36.3259, 24.6825) projected
  line L205 (-36.3259, 24.6825) -> (-24.7508, 13.1453) projected
  line L206 (-24.7508, 13.1453) -> (-26.5571, 11.3331) projected
  line L207 (-30.2744, 3.2872) -> (-32.0676, 5.1044) projected
  line L208 (-32.0676, 5.1044) -> (-26.5973, 10.5022) projected
  line L209 (-26.5973, 10.5022) -> (-24.8042, 8.6849) projected
  line L210 (-24.8042, 8.6849) -> (-30.2744, 3.2872) projected
  line L211 (-33.3036, 13.605) -> (-40.3585, 20.6367) projected
  line L212 (-40.3585, 20.6367) -> (-38.5432, 22.458) projected
  line L213 (-38.5432, 22.458) -> (-31.4884, 15.4262) projected
  line L214 (-31.4884, 15.4262) -> (-33.3036, 13.605) projected
  line L215 (-54.0136, -35.0444) -> (-39.4592, -31.4155) projected
  line L216 (-39.4592, -31.4155) -> (-35.8303, -45.97) projected
  line L217 (-35.8303, -45.97) -> (-50.3848, -49.5988) projected
  line L218 (-50.3848, -49.5988) -> (-54.0136, -35.0444) projected
  line L219 (-67.7189, -18.1574) -> (-56.5717, -8.1205) projected
  line L220 (-56.5717, -8.1205) -> (-46.5348, -19.2676) projected
  line L221 (-46.5348, -19.2676) -> (-57.682, -29.3046) projected
  line L222 (-57.682, -29.3046) -> (-67.7189, -18.1574) projected
  line L223 (-9.4622, -31.4155) -> (5.0923, -35.0444) projected
  line L224 (5.0923, -35.0444) -> (1.4635, -49.5988) projected
  line L225 (1.4635, -49.5988) -> (-13.091, -45.97) projected
  line L226 (-13.091, -45.97) -> (-9.4622, -31.4155) projected
  line L227 (7.6504, -8.1205) -> (18.7976, -18.1574) projected
  line L228 (18.7976, -18.1574) -> (8.7607, -29.3046) projected
  line L229 (8.7607, -29.3046) -> (-2.3865, -19.2676) projected
  line L230 (-2.3865, -19.2676) -> (7.6504, -8.1205) projected
  line L231 (-111.5432, 80.9928) -> (-91.8441, 81.9679) projected
  line L232 (-90.6697, 81.7906) -> (-70.2485, 74.3579) projected
  line L233 (-137.7551, 74.6394) -> (-112.0999, 80.9125) projected
  line L234 (-154.4405, 18.3871) -> (-139.9403, 72.5018) projected
  line L235 (-134.0073, 9.8061) -> (-152.319, 14.7128) projected
  line L236 (-111.9401, 15.8297) -> (-132.3855, 9.8255) projected
  line L237 (-98.1783, 13.1596) -> (-110.4455, 15.8801) projected
  line L238 (-92.4348, -9.3825) -> (-95.8914, 10.7429) projected
  line L239 (-74.5563, -17.3936) -> (-90.4875, -11.6997) projected
  line L240 (-58.4773, -34.2497) -> (-72.7201, -18.4315) projected
  line L241 (-53.938, -51.3943) -> (-57.7859, -35.5723) projected
  line L242 (-31.4601, -48.8997) -> (-50.2976, -53.5965) projected
  line L243 (-18.187, -48.8106) -> (-30.7343, -48.8106) projected
  line L244 (-17.4612, -48.8997) -> (1.3763, -53.5965) projected
  line L245 (5.0167, -51.3943) -> (8.8645, -35.5723) projected
  line L246 (9.556, -34.2497) -> (23.7988, -18.4315) projected
  line L247 (25.635, -17.3936) -> (41.5662, -11.6997) projected
  line L248 (43.5135, -9.3825) -> (46.9701, 10.7429) projected
  line L249 (49.257, 13.1596) -> (61.5242, 15.8801) projected
  line L250 (63.0188, 15.8297) -> (83.4642, 9.8255) projected
  line L251 (85.086, 9.8061) -> (103.3977, 14.7128) projected
  line L252 (105.5192, 18.3871) -> (91.019, 72.5018) projected
  line L253 (88.8338, 74.6394) -> (63.1786, 80.9125) projected
  line L254 (62.6219, 80.9928) -> (42.9227, 81.9679) projected
  line L255 (41.7484, 81.7906) -> (21.3272, 74.3579) projected
  line L256 (20.5259, 73.9182) -> (5.3305, 62.2476) projected
  line L257 (4.8188, 61.9306) -> (-10.8605, 54.2803) projected
  line L258 (-12.7723, 53.6855) -> (-24.4607, 53.6855) projected
  line L259 (-36.149, 53.6855) -> (-24.4607, 53.6855) projected
  line L260 (-53.7401, 61.9306) -> (-38.0608, 54.2803) projected
  line L261 (-69.4472, 73.9182) -> (-54.2518, 62.2476) projected
  arc A29 (-137.7551, 74.6394) -> (-139.9403, 72.5018) centre (-137.0425, 71.7251) ccw
  arc A30 (-154.4405, 18.3871) -> (-152.319, 14.7128) centre (-151.5428, 17.6106) ccw
  arc A31 (-134.0073, 9.8061) -> (-132.3855, 9.8255) centre (-133.2309, 12.7035) ccw
  arc A32 (-95.8914, 10.7429) -> (-98.1783, 13.1596) centre (-98.8211, 10.2609) ccw
  arc A33 (-92.4348, -9.3825) -> (-90.4875, -11.6997) centre (-89.4782, -8.8747) ccw
  arc A34 (-72.7201, -18.4315) -> (-74.5563, -17.3936) centre (-76.6396, -23.2223) ccw
  arc A35 (-57.7859, -35.5723) -> (-58.4773, -34.2497) centre (-60.7074, -36.2577) ccw
  arc A36 (-53.938, -51.3943) -> (-50.2976, -53.5965) centre (-51.0229, -50.6854) ccw
  arc A37 (-30.7343, -48.8106) -> (-31.4601, -48.8997) centre (-30.7343, -51.8105) ccw
  arc A38 (-17.4612, -48.8997) -> (-18.187, -48.8106) centre (-18.187, -51.8105) ccw
  arc A39 (1.3763, -53.5965) -> (5.0167, -51.3943) centre (2.1019, -50.686) ccw
  arc A40 (9.556, -34.2497) -> (8.8645, -35.5723) centre (11.8759, -36.3046) ccw
  arc A41 (25.635, -17.3936) -> (23.7988, -18.4315) centre (26.2659, -20.6529) ccw
  arc A42 (41.5662, -11.6997) -> (43.5135, -9.3825) centre (40.5563, -8.8742) ccw
  arc A43 (49.257, 13.1596) -> (46.9701, 10.7429) centre (49.9272, 10.235) ccw
  arc A44 (63.0188, 15.8297) -> (61.5242, 15.8801) centre (62.1736, 12.9516) ccw
  arc A45 (83.4642, 9.8255) -> (85.086, 9.8061) centre (84.3096, 12.7044) ccw
  arc A46 (103.3977, 14.7128) -> (105.5192, 18.3871) centre (102.6211, 17.6108) ccw
  arc A47 (91.019, 72.5018) -> (88.8338, 74.6394) centre (88.1214, 71.7253) ccw
  arc A48 (63.1786, 80.9125) -> (62.6219, 80.9928) centre (62.4855, 78.0777) ccw
  arc A49 (42.9227, 81.9679) -> (41.7484, 81.7906) centre (42.7745, 78.9724) ccw
  arc A50 (21.3272, 74.3579) -> (20.5259, 73.9182) centre (22.3538, 71.5374) ccw
  arc A51 (4.8188, 61.9306) -> (5.3305, 62.2476) centre (3.5014, 64.629) ccw
  arc A52 (-12.7723, 53.6855) -> (-10.8605, 54.2803) centre (-13.7536, 60.2096) ccw
  arc A53 (-38.0608, 54.2803) -> (-36.149, 53.6855) centre (-36.149, 57.0556) ccw
  arc A54 (-54.2518, 62.2476) -> (-53.7401, 61.9306) centre (-52.4258, 64.6241) ccw
  arc A55 (-69.4472, 73.9182) -> (-70.2485, 74.3579) centre (-71.2736, 71.5402) ccw
  arc A56 (-90.6697, 81.7906) -> (-91.8441, 81.9679) centre (-91.696, 78.9707) ccw
  arc A57 (-111.5432, 80.9928) -> (-112.0999, 80.9125) centre (-111.3949, 77.9952) ccw
  arc A58 (-110.4455, 15.8801) -> (-111.9401, 15.8297) centre (-111.0949, 12.9519) ccw
  point P0 (0, 0)
  constraints: 60 point on circle, 31 tangent, 30 centre point
ref_plane "Arbeitsebene1" through (-107.6215, -19.2336, -6.6) normal (0, 0, -1) x (0, 1, 0)
extrude "Extrusion3" add sketch "Skizze5" along normal up to surface (5.1 mm away) contours A27 L30 A26 L29 A25 L28 A24 L27 A23 L26 A22 L25 L24 A21 L23 A20 L22 L21 L20 A19 L19 A18 L18 A17 L17 A16 L16 A15 L15 A14 L14 A13 L13 A12 L12 A11 L11 A10 L10 A9 L9 A8 L8 A7 L7 A6 L6 A5 L5 A4 L4 A3 L3 A2 L2 A1 L1 A0 L0